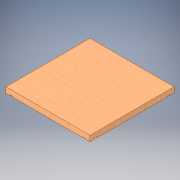
# Autodesk Inventor part: Bauteil3
Saved by Autodesk Inventor 2019.5 (Build 235369000, 369)
## iProperties
Created: 2021-09-27
Part Number: Bauteil3
Material: Holz (Kirsche)
Document SubType Name: Modeling
Designer: mritt
Density: 0.63 g/cm^3
Appearance: Kirsche - natur - schwacher Glanz
Mass: 1130.89 g
Surface Area: 2053.78 cm^2
Volume: 1795.07 cm^3
Author: mritt
Autodesk Inventor part; units mm, degrees
ref_plane "YZ Plane" through (0, 0, 0) normal (1, 0, 0) x (0, 1, 0)
ref_plane "XZ Plane" through (0, 0, 0) normal (0, 1, 0) x (-1, 0, 0)
ref_plane "XY Plane" through (0, 0, 0) normal (0, 0, 1) x (1, 0, 0)
sketch "Skizze1" plane through (0, 0, 0) normal (0, 1, 0) x (-1, 0, 0)
  line L0 (387.1429, -272.5) -> (87.1429, -272.5)
  line L1 (87.1429, -272.5) -> (87.1429, -572.5)
  line L2 (87.1429, -572.5) -> (387.1429, -572.5)
  line L3 (387.1429, -572.5) -> (387.1429, -272.5)
  circle A0 centre (107.1429, -292.5) radius 3.75
  circle A1 centre (367.1429, -292.5) radius 3.75
  circle A2 centre (367.1429, -552.5) radius 3.75
  circle A3 centre (107.1429, -552.5) radius 3.75
  line L4 (387.1429, -297.5) -> (362.1429, -297.5)
  line L5 (362.1429, -297.5) -> (362.1429, -287.5)
  line L6 (362.1429, -287.5) -> (387.1429, -287.5)
  line L7 (387.1429, -287.5) -> (387.1429, -297.5)
  line L8 (362.1429, -272.5) -> (372.1429, -272.5)
  line L9 (372.1429, -272.5) -> (372.1429, -297.5)
  line L10 (372.1429, -297.5) -> (362.1429, -297.5)
  line L11 (362.1429, -297.5) -> (362.1429, -272.5)
  line L12 (362.1429, -572.5) -> (372.1429, -572.5)
  line L13 (372.1429, -572.5) -> (372.1429, -547.5)
  line L14 (372.1429, -547.5) -> (362.1429, -547.5)
  line L15 (362.1429, -547.5) -> (362.1429, -572.5)
  line L16 (387.1429, -547.5) -> (362.1429, -547.5)
  line L17 (362.1429, -547.5) -> (362.1429, -557.5)
  line L18 (362.1429, -557.5) -> (387.1429, -557.5)
  line L19 (387.1429, -557.5) -> (387.1429, -547.5)
  line L20 (112.1429, -547.5) -> (87.1429, -547.5)
  line L21 (87.1429, -547.5) -> (87.1429, -557.5)
  line L22 (87.1429, -557.5) -> (112.1429, -557.5)
  line L23 (112.1429, -557.5) -> (112.1429, -547.5)
  line L24 (112.1429, -547.5) -> (102.1429, -547.5)
  line L25 (102.1429, -547.5) -> (102.1429, -572.5)
  line L26 (102.1429, -572.5) -> (112.1429, -572.5)
  line L27 (112.1429, -572.5) -> (112.1429, -547.5)
  line L28 (112.1429, -287.5) -> (87.1429, -287.5)
  line L29 (87.1429, -287.5) -> (87.1429, -297.5)
  line L30 (87.1429, -297.5) -> (112.1429, -297.5)
  line L31 (112.1429, -297.5) -> (112.1429, -287.5)
  line L32 (112.1429, -297.5) -> (102.1429, -297.5)
  line L33 (102.1429, -297.5) -> (102.1429, -272.5)
  line L34 (102.1429, -272.5) -> (112.1429, -272.5)
  line L35 (112.1429, -272.5) -> (112.1429, -297.5)
  circle A4 centre (367.1429, -552.5) radius 5
  circle A5 centre (107.1429, -552.5) radius 5
  circle A6 centre (107.1429, -292.5) radius 5
  circle A7 centre (367.1429, -292.5) radius 5
  point P0 (0, 0)
  dimension "d0" = 300
  dimension "d1" = 300
  dimension "d2" = 7.5
  dimension "d3" = 7.5
  dimension "d4" = 7.5
  dimension "d5" = 7.5
  dimension "d6" = 20
  dimension "d7" = 20
  dimension "d8" = 20
  dimension "d9" = 20
  dimension "d10" = 20
  dimension "d12" = 20
  dimension "d13" = 20
  dimension "d23" = 10
  dimension "d24" = 10
  dimension "d25" = 25
  dimension "d26" = 25
  dimension "d27" = 25
  dimension "d28" = 25
  dimension "d29" = 25
  dimension "d30" = 25
  dimension "d31" = 10
  dimension "d32" = 10
  dimension "d33" = 10
  dimension "d34" = 10
  dimension "d35" = 10
  dimension "d36" = 10
  dimension "d37" = 10
  dimension "d38" = 10
  constraints: 72 end point, 18 parallel, 16 point on line, 9 horizontal, 9 perpendicular, 8 centre point, 4 coincident
  measures "d0" distance of L1.end L2.end
  measures "d1" distance of L0.end L1.end
  measures "d2" diameter of A0
  measures "d3" diameter of A3
  measures "d4" diameter of A2
  measures "d5" diameter of A1
  measures "d6" distance from line of A0.centre L0
  measures "d7" distance from line of A0.centre L1
  measures "d8" distance from line of A1.centre L0
  measures "d9" distance from line of A2.centre L3
  measures "d10" distance from line of A1.centre L3
  measures "d12" distance from line of A3.centre L2
  measures "d13" distance from line of A3.centre L1
  measures "d23" distance between parallel lines of L30 L28
  measures "d24" distance between parallel lines of L33 L35
  measures "d25" distance of L34.end L30.end
  measures "d26" distance of L29.end L30.end
  measures "d27" distance of L26.end L20.start
  measures "d28" distance of L16.start L16.end
  measures "d29" distance of L10.end L8.start
  measures "d30" distance of L4.start L4.end
  measures "d31" distance between parallel lines of L15 L13
  measures "d32" distance between parallel lines of L22 L20
  measures "d33" distance between parallel lines of L11 L9
  measures "d34" distance between parallel lines of L6 L4
  measures "d35" diameter of A4
  measures "d36" diameter of A5
  measures "d37" diameter of A6
  measures "d38" diameter of A7
extrude "Extrusion1" add sketch "Skizze1" along normal blind 20 contours L3 L6 L9 L0 | L9 L6 L11 L0 | L3 L4 L9 L6 | L11 L5 L4 L3 L16 L14 L15 L2 L27 L23 L20 L1 L30 L31 L35 L0 | L9 A7 L6 | L35 L28 L33 L0 | L6 A7 L5 | A7 | L9 L4 A7 | L3 L18 L13 L16 | L33 L28 L1 L0 | L31 A6 L28 | A7 L4 L5 | L3 L2 L13 L18 | L13 A4 L14 | L33 L30 L1 L28 | L28 A6 L33 | A6 | L31 L30 A6 | L18 A4 L13 | L13 L2 L15 L18 | A4 | A4 L15 L14 | A6 L30 L33 | L18 L15 A4 | L20 L25 L22 L1 | L2 L25 L22 L27 | L22 L25 L2 L1 | L20 A5 L25 | L22 A5 L23 | L25 A5 L22 | L20 L23 A5 | A5 | A0 | A1 | A2 | A3
extrude "Extrusion2" cut sketch "Skizze1" along normal blind 3 contours L9 L6 L11 L0 | L3 L4 L9 L6 | L9 A7 L6 | L35 L28 L33 L0 | L6 A7 L5 | A7 | L9 L4 A7 | L3 L18 L13 L16 | L31 A6 L28 | A7 L4 L5 | L13 A4 L14 | L33 L30 L1 L28 | L28 A6 L33 | A6 | L31 L30 A6 | L18 A4 L13 | L13 L2 L15 L18 | A4 | A4 L15 L14 | A6 L30 L33 | L18 L15 A4 | L20 L25 L22 L1 | L2 L25 L22 L27 | L20 A5 L25 | L22 A5 L23 | L25 A5 L22 | L20 L23 A5 | A5 | A0 | A1 | A2 | A3
extrude "Extrusion3" cut sketch "Skizze1" along normal blind 10 contours A0 | A1 | A2 | A3
extrude "Extrusion4" cut sketch "Skizze1" along normal blind 6 contours A7 | A6 | A4 | A5
